Autodesk Inventor part; units mm, degrees
(part 4 of 5)
  spline S23 degree 5 poles (4.4219, -3.499) (4.422, -3.499) (4.4221, -3.4991) (4.4222, -3.4992) (4.4225, -3.4994) (4.423, -3.4998) (4.4234, -3.5001) (4.424, -3.5005) (4.4246, -3.501) (4.4253, -3.5015) (4.426, -3.502) (4.4268, -3.5026) (4.4277, -3.5032) (4.4286, -3.5039) (4.4296, -3.5046) (4.4307, -3.5053) (4.4318, -3.5061) (4.433, -3.5069) (4.4342, -3.5077) (4.4355, -3.5086) (4.4369, -3.5095) (4.4383, -3.5104) (4.4398, -3.5114) (4.4413, -3.5124) (4.4429, -3.5135) (4.4446, -3.5145) (4.4463, -3.5156) (4.4481, -3.5168) (4.4499, -3.5179) (4.4518, -3.5191) (4.4538, -3.5203) (4.4558, -3.5215) (4.4583, -3.5231) (4.4609, -3.5246) (4.4635, -3.5262) (4.4667, -3.5281) (4.4701, -3.53) (4.473, -3.5317) (4.4765, -3.5337) (4.4802, -3.5358) (4.4834, -3.5376) (4.4867, -3.5394) (4.4906, -3.5416) (4.4958, -3.5444) (4.5012, -3.5473) (4.5068, -3.5502) (4.5125, -3.5532) (4.5185, -3.5562) (4.5232, -3.5586) (4.528, -3.561) (4.533, -3.5635) (4.5387, -3.5663) (4.5439, -3.5687) (4.5484, -3.5709) (4.5538, -3.5734) (4.5592, -3.5759) (4.564, -3.5781) (4.5696, -3.5807) (4.5753, -3.5832) (4.5803, -3.5855) (4.5862, -3.5881) (4.5923, -3.5907) (4.5975, -3.5929) (4.6037, -3.5955) (4.61, -3.5982) (4.6155, -3.6004) (4.6219, -3.6031) (4.6285, -3.6057) (4.6342, -3.608) (4.641, -3.6107) (4.6478, -3.6133) (4.6537, -3.6156) (4.6607, -3.6183) (4.6679, -3.6209) (4.674, -3.6232) (4.6813, -3.6259) (4.6887, -3.6285) (4.6951, -3.6308) (4.7026, -3.6335) (4.7102, -3.6361) (4.7168, -3.6384) (4.7246, -3.641) (4.7325, -3.6437) (4.7393, -3.6459) (4.7474, -3.6485) (4.7555, -3.6511) (4.7626, -3.6533) (4.7708, -3.6559) (4.7792, -3.6585) (4.7865, -3.6607) (4.795, -3.6632) (4.8036, -3.6658) (4.8111, -3.6679) (4.8199, -3.6705) (4.8288, -3.6729) (4.8364, -3.6751) (4.8454, -3.6775) (4.8545, -3.68) (4.8624, -3.6821) (4.8717, -3.6845) (4.881, -3.6869) (4.8891, -3.6889) (4.8985, -3.6912) (4.9081, -3.6936) (4.9164, -3.6956) (4.9261, -3.6978) (4.9359, -3.7001) (4.9443, -3.702) (4.9543, -3.7043) (4.9643, -3.7065) (4.9729, -3.7083) (4.9831, -3.7105) (4.9933, -3.7126) (5.0021, -3.7144) (5.0125, -3.7165) (5.023, -3.7185) (5.032, -3.7202) (5.0425, -3.7222) (5.0532, -3.7242) (5.0624, -3.7258) (5.0732, -3.7277) (5.0841, -3.7296) (5.0934, -3.7312) (5.1044, -3.733) (5.1155, -3.7348) (5.1251, -3.7363) (5.1363, -3.738) (5.1475, -3.7397) (5.1572, -3.7411) (5.1686, -3.7427) (5.1801, -3.7443) (5.19, -3.7456) (5.2016, -3.7472) (5.2133, -3.7486) (5.2233, -3.7499) (5.2351, -3.7513) (5.247, -3.7527) (5.2572, -3.7538) (5.2692, -3.7551) (5.2812, -3.7564) (5.2916, -3.7574) (5.3037, -3.7586) (5.316, -3.7598) (5.3265, -3.7607) (5.3388, -3.7618) (5.3513, -3.7628) (5.3619, -3.7637) (5.3763, -3.7648) (5.3907, -3.7658) (5.4033, -3.7667) (5.4161, -3.7675) (5.4289, -3.7682) (5.4435, -3.7691) (5.4583, -3.7698) (5.4731, -3.7705) (5.4881, -3.7712) (5.505, -3.7718) (5.5163, -3.7722) (5.5276, -3.7726) (5.5428, -3.773) (5.5581, -3.7734) (5.5715, -3.7736) (5.585, -3.7738) (5.5985, -3.774) (5.6082, -3.7741) (5.6179, -3.7741) (5.6277, -3.7742) (5.6375, -3.7742) (5.6473, -3.7742) (5.6571, -3.7742) (5.667, -3.7741) (5.6769, -3.774) (5.6868, -3.7739) (5.6967, -3.7738) (5.7067, -3.7736) (5.7167, -3.7734) (5.7267, -3.7732) (5.7368, -3.7729) (5.7468, -3.7727) (5.757, -3.7724) (5.7671, -3.772) (5.7772, -3.7717) (5.7874, -3.7713) (5.7976, -3.7709) (5.8079, -3.7705) (5.8181, -3.77) (5.8284, -3.7695) (5.8387, -3.769) (5.849, -3.7685) (5.8635, -3.7677) (5.876, -3.7669) (5.8864, -3.7663) (5.8948, -3.7657) (5.901, -3.7653) knots 0 0 0 0 0 0 0.004167 0.008333 0.0125 0.016667 0.020833 0.025 0.029167 0.033333 0.0375 0.041667 0.045833 0.05 0.054167 0.058333 0.0625 0.066667 0.070833 0.075 0.079167 0.083333 0.0875 0.091667 0.095833 0.1 0.104167 0.108333 0.1125 0.116667 0.120833 0.125 0.129167 0.1375 0.141667 0.145833 0.154167 0.158333 0.1625 0.170833 0.175 0.179167 0.183333 0.191667 0.208333 0.2125 0.216667 0.220833 0.229167 0.2375 0.241667 0.245833 0.254167 0.258333 0.2625 0.270833 0.275 0.279167 0.2875 0.291667 0.295833 0.304167 0.308333 0.3125 0.320833 0.325 0.329167 0.3375 0.341667 0.345833 0.354167 0.358333 0.3625 0.370833 0.375 0.379167 0.3875 0.391667 0.395833 0.404167 0.408333 0.4125 0.420833 0.425 0.429167 0.4375 0.441667 0.445833 0.454167 0.458333 0.4625 0.470833 0.475 0.479167 0.4875 0.491667 0.495833 0.504167 0.508333 0.5125 0.520833 0.525 0.529167 0.5375 0.541667 0.545833 0.554167 0.558333 0.5625 0.570833 0.575 0.579167 0.5875 0.591667 0.595833 0.604167 0.608333 0.6125 0.620833 0.625 0.629167 0.6375 0.641667 0.645833 0.654167 0.658333 0.6625 0.670833 0.675 0.679167 0.6875 0.691667 0.695833 0.704167 0.708333 0.7125 0.720833 0.725 0.729167 0.7375 0.741667 0.745833 0.754167 0.758333 0.7625 0.770833 0.775 0.779167 0.791667 0.795833 0.8 0.804167 0.808333 0.825 0.829167 0.833333 0.8375 0.845833 0.85 0.854167 0.866667 0.870833 0.875 0.879167 0.883333 0.8875 0.891667 0.895833 0.9 0.904167 0.908333 0.9125 0.916667 0.920833 0.925 0.929167 0.933333 0.9375 0.941667 0.945833 0.95 0.954167 0.958333 0.9625 0.966667 0.970833 0.975 0.979167 0.983333 0.9875 1 1 1 1 1 1
  arc A23 (5.901, -3.7653) -> (6.2114, -3.2278) centre (0, 0) ccw
  circle A24 centre (0, 0) radius 3 construction
  line L24 (-4.4832, 3.4199) -> (-3.7077, 2.8063)
  arc A25 (-2.8063, 3.7077) -> (-3.7077, 2.8063) centre (0, 0) ccw
  line L25 (-2.8063, 3.7077) -> (-3.4199, 4.4832)
  arc A26 (-3.2267, 6.0991) -> (-3.6686, 5.8439) centre (0, 0) ccw
  line L26 (-2.1726, 5.2033) -> (-1.8078, 4.2842)
  arc A27 (-0.5765, 4.6141) -> (-1.8078, 4.2842) centre (0, 0) ccw
  line L27 (-0.5765, 4.6141) -> (-0.7202, 5.5925)
  arc A28 (0.2551, 6.8953) -> (-0.2551, 6.8953) centre (0, 0) ccw
  line L28 (0.7202, 5.5925) -> (0.5765, 4.6141)
  arc A29 (1.8078, 4.2842) -> (0.5765, 4.6141) centre (0, 0) ccw
  line L29 (1.8078, 4.2842) -> (2.1726, 5.2033)
  arc A30 (3.6686, 5.8439) -> (3.2267, 6.0991) centre (0, 0) ccw
  line L30 (3.4199, 4.4832) -> (2.8063, 3.7077)
  arc A31 (3.7077, 2.8063) -> (2.8063, 3.7077) centre (0, 0) ccw
  line L31 (3.7077, 2.8063) -> (4.4832, 3.4199)
  arc A32 (6.0991, 3.2267) -> (5.8439, 3.6686) centre (0, 0) ccw
  line L32 (5.2033, 2.1726) -> (4.2842, 1.8078)
  arc A33 (4.6141, 0.5765) -> (4.2842, 1.8078) centre (0, 0) ccw
  line L33 (4.6141, 0.5765) -> (5.5925, 0.7202)
  arc A34 (6.8953, -0.2551) -> (6.8953, 0.2551) centre (0, 0) ccw
  line L34 (5.5925, -0.7202) -> (4.6141, -0.5765)
  arc A35 (4.2842, -1.8078) -> (4.6141, -0.5765) centre (0, 0) ccw
  line L35 (4.2842, -1.8078) -> (5.2033, -2.1726)
  arc A36 (5.8439, -3.6686) -> (6.0991, -3.2267) centre (0, 0) ccw
  line L36 (4.4832, -3.4199) -> (3.7077, -2.8063)
  arc A37 (2.8063, -3.7077) -> (3.7077, -2.8063) centre (0, 0) ccw
  line L37 (2.8063, -3.7077) -> (3.4199, -4.4832)
  arc A38 (3.2267, -6.0991) -> (3.6686, -5.8439) centre (0, 0) ccw
  line L38 (2.1726, -5.2033) -> (1.8078, -4.2842)
  arc A39 (0.5765, -4.6141) -> (1.8078, -4.2842) centre (0, 0) ccw
  line L39 (0.5765, -4.6141) -> (0.7202, -5.5925)
  arc A40 (-0.2551, -6.8953) -> (0.2551, -6.8953) centre (0, 0) ccw
  line L40 (-0.7202, -5.5925) -> (-0.5765, -4.6141)
  arc A41 (-1.8078, -4.2842) -> (-0.5765, -4.6141) centre (0, 0) ccw
  line L41 (-1.8078, -4.2842) -> (-2.1726, -5.2033)
  arc A42 (-3.6686, -5.8439) -> (-3.2267, -6.0991) centre (0, 0) ccw
  line L42 (-3.4199, -4.4832) -> (-2.8063, -3.7077)
  arc A43 (-3.7077, -2.8063) -> (-2.8063, -3.7077) centre (0, 0) ccw
  line L43 (-3.7077, -2.8063) -> (-4.4832, -3.4199)
  arc A44 (-6.0991, -3.2267) -> (-5.8439, -3.6686) centre (0, 0) ccw
  line L44 (-5.2033, -2.1726) -> (-4.2842, -1.8078)
  arc A45 (-4.6141, -0.5765) -> (-4.2842, -1.8078) centre (0, 0) ccw
  line L45 (-4.6141, -0.5765) -> (-5.5925, -0.7202)
  arc A46 (-6.8953, 0.2551) -> (-6.8953, -0.2551) centre (0, 0) ccw
  line L46 (-5.5925, 0.7202) -> (-4.6141, 0.5765)
  arc A47 (-4.2842, 1.8078) -> (-4.6141, 0.5765) centre (0, 0) ccw
  line L47 (-4.2842, 1.8078) -> (-5.2033, 2.1726)
  arc A48 (-5.8439, 3.6686) -> (-6.0991, 3.2267) centre (0, 0) ccw
  line L48 (-0.5765, 4.6141) -> (0.5765, 4.6141) construction
  spline S24 degree 5 poles (-3.4199, 4.4832) (-3.4189, 4.4818) (-3.4217, 4.4856) (-3.4213, 4.485) (-3.4244, 4.4895) (-3.4266, 4.4928) (-3.4288, 4.496) (-3.4335, 4.5035) (-3.4383, 4.5113) (-3.4411, 4.5161) (-3.4477, 4.5274) (-3.454, 4.5388) (-3.4576, 4.5454) (-3.4654, 4.5602) (-3.4728, 4.5752) (-3.4769, 4.5835) (-3.4855, 4.6017) (-3.4937, 4.62) (-3.4981, 4.63) (-3.5072, 4.6514) (-3.5159, 4.673) (-3.5204, 4.6845) (-3.5297, 4.709) (-3.5385, 4.7337) (-3.543, 4.7467) (-3.5522, 4.7741) (-3.5609, 4.8017) (-3.5653, 4.8162) (-3.5742, 4.8465) (-3.5825, 4.8769) (-3.5867, 4.8927) (-3.5951, 4.9256) (-3.6028, 4.9587) (-3.6067, 4.9758) (-3.6144, 5.0113) (-3.6214, 5.0469) (-3.6248, 5.0653) (-3.6316, 5.1033) (-3.6377, 5.1413) (-3.6407, 5.1609) (-3.6464, 5.2011) (-3.6514, 5.2414) (-3.6538, 5.2621) (-3.6584, 5.3045) (-3.6622, 5.347) (-3.664, 5.3688) (-3.6673, 5.4132) (-3.6698, 5.4578) (-3.6708, 5.4805) (-3.6727, 5.527) (-3.6737, 5.5734) (-3.6741, 5.5971) (-3.6744, 5.6454) (-3.6739, 5.6937) (-3.6735, 5.7183) (-3.6724, 5.7581) (-3.6708, 5.798) (-3.6702, 5.8133) (-3.6694, 5.8286) (-3.6686, 5.8439) knots 0 0 0 0 0 0 0.004377 0.004377 0.004377 0.016733 0.016733 0.016733 0.036594 0.036594 0.036594 0.063277 0.063277 0.063277 0.096218 0.096218 0.096218 0.134948 0.134948 0.134948 0.179064 0.179064 0.179064 0.228222 0.228222 0.228222 0.282124 0.282124 0.282124 0.340507 0.340507 0.340507 0.403138 0.403138 0.403138 0.46981 0.46981 0.46981 0.540337 0.540337 0.540337 0.614551 0.614551 0.614551 0.692299 0.692299 0.692299 0.773444 0.773444 0.773444 0.857857 0.857857 0.857857 0.945422 0.945422 0.945422 1 1 1 1 1 1
  spline S25 degree 5 poles (-3.2267, 6.0991) (-3.213, 6.0921) (-3.1994, 6.0851) (-3.1858, 6.078) (-3.1505, 6.0595) (-3.1154, 6.0404) (-3.0939, 6.0285) (-3.0519, 6.0048) (-3.0102, 5.9804) (-2.9899, 5.9683) (-2.9502, 5.9441) (-2.9109, 5.9193) (-2.8917, 5.907) (-2.8544, 5.8826) (-2.8175, 5.8575) (-2.7995, 5.8451) (-2.7646, 5.8205) (-2.7302, 5.7954) (-2.7135, 5.7829) (-2.6811, 5.7584) (-2.6491, 5.7333) (-2.6336, 5.721) (-2.6037, 5.6967) (-2.5743, 5.6719) (-2.5601, 5.6597) (-2.5328, 5.6358) (-2.5059, 5.6114) (-2.4929, 5.5995) (-2.4682, 5.5762) (-2.4439, 5.5525) (-2.4322, 5.541) (-2.4101, 5.5186) (-2.3883, 5.4957) (-2.378, 5.4847) (-2.3584, 5.4634) (-2.3393, 5.4417) (-2.3302, 5.4312) (-2.3133, 5.4113) (-2.2967, 5.391) (-2.289, 5.3813) (-2.2746, 5.363) (-2.2607, 5.3444) (-2.2542, 5.3357) (-2.2424, 5.3194) (-2.231, 5.3028) (-2.2258, 5.2952) (-2.2166, 5.2812) (-2.2077, 5.2671) (-2.2037, 5.2607) (-2.197, 5.2495) (-2.1905, 5.2381) (-2.1878, 5.2334) (-2.1834, 5.2252) (-2.1793, 5.2174) (-2.1776, 5.2139) (-2.1758, 5.2104) (-2.1735, 5.2054) (-2.1738, 5.2061) (-2.1719, 5.2017) (-2.1726, 5.2033) knots 0 0 0 0 0 0 0.054578 0.054578 0.054578 0.142143 0.142143 0.142143 0.226556 0.226556 0.226556 0.307701 0.307701 0.307701 0.385449 0.385449 0.385449 0.459663 0.459663 0.459663 0.53019 0.53019 0.53019 0.596862 0.596862 0.596862 0.659493 0.659493 0.659493 0.717876 0.717876 0.717876 0.771778 0.771778 0.771778 0.820936 0.820936 0.820936 0.865052 0.865052 0.865052 0.903782 0.903782 0.903782 0.936723 0.936723 0.936723 0.963406 0.963406 0.963406 0.983267 0.983267 0.983267 0.995623 0.995623 0.995623 1 1 1 1 1 1
  spline S26 degree 5 poles (-0.7202, 5.5925) (-0.7199, 5.5908) (-0.7205, 5.5955) (-0.7204, 5.5948) (-0.7209, 5.6002) (-0.7211, 5.6042) (-0.7214, 5.6081) (-0.7218, 5.6169) (-0.722, 5.6261) (-0.7221, 5.6316) (-0.7221, 5.6447) (-0.7219, 5.6577) (-0.7216, 5.6652) (-0.721, 5.6819) (-0.72, 5.6987) (-0.7193, 5.7079) (-0.7177, 5.7279) (-0.7157, 5.7479) (-0.7144, 5.7588) (-0.7116, 5.7818) (-0.7083, 5.8049) (-0.7065, 5.8171) (-0.7023, 5.843) (-0.6976, 5.8687) (-0.695, 5.8823) (-0.6892, 5.9106) (-0.683, 5.9389) (-0.6795, 5.9536) (-0.6721, 5.9842) (-0.6641, 6.0147) (-0.6598, 6.0306) (-0.6506, 6.0632) (-0.6408, 6.0958) (-0.6356, 6.1126) (-0.6245, 6.1471) (-0.6127, 6.1815) (-0.6065, 6.1991) (-0.5934, 6.2353) (-0.5797, 6.2713) (-0.5725, 6.2898) (-0.5573, 6.3275) (-0.5415, 6.3649) (-0.5333, 6.384) (-0.516, 6.423) (-0.4981, 6.4618) (-0.4887, 6.4815) (-0.4693, 6.5216) (-0.4492, 6.5615) (-0.4388, 6.5817) (-0.4172, 6.6228) (-0.3948, 6.6636) (-0.3833, 6.6843) (-0.3594, 6.7263) (-0.3349, 6.7678) (-0.3222, 6.7889) (-0.3013, 6.8229) (-0.28, 6.8567) (-0.2718, 6.8696) (-0.2635, 6.8824) (-0.2551, 6.8953) knots 0 0 0 0 0 0 0.004377 0.004377 0.004377 0.016733 0.016733 0.016733 0.036594 0.036594 0.036594 0.063277 0.063277 0.063277 0.096218 0.096218 0.096218 0.134948 0.134948 0.134948 0.179064 0.179064 0.179064 0.228222 0.228222 0.228222 0.282124 0.282124 0.282124 0.340507 0.340507 0.340507 0.403138 0.403138 0.403138 0.46981 0.46981 0.46981 0.540337 0.540337 0.540337 0.614551 0.614551 0.614551 0.692299 0.692299 0.692299 0.773444 0.773444 0.773444 0.857857 0.857857 0.857857 0.945422 0.945422 0.945422 1 1 1 1 1 1
  spline S27 degree 5 poles (0.2551, 6.8953) (0.2635, 6.8824) (0.2718, 6.8696) (0.28, 6.8567) (0.3013, 6.8229) (0.3222, 6.7889) (0.3349, 6.7678) (0.3594, 6.7263) (0.3833, 6.6843) (0.3948, 6.6636) (0.4172, 6.6228) (0.4388, 6.5817) (0.4492, 6.5615) (0.4693, 6.5216) (0.4887, 6.4815) (0.4981, 6.4618) (0.516, 6.423) (0.5333, 6.384) (0.5415, 6.3649) (0.5573, 6.3275) (0.5725, 6.2898) (0.5797, 6.2713) (0.5934, 6.2353) (0.6065, 6.1991) (0.6127, 6.1815) (0.6245, 6.1471) (0.6356, 6.1126) (0.6408, 6.0958) (0.6506, 6.0632) (0.6598, 6.0306) (0.6641, 6.0147) (0.6721, 5.9842) (0.6795, 5.9536) (0.683, 5.9389) (0.6892, 5.9106) (0.695, 5.8823) (0.6976, 5.8687) (0.7023, 5.843) (0.7065, 5.8171) (0.7083, 5.8049) (0.7116, 5.7818) (0.7144, 5.7588) (0.7157, 5.7479) (0.7177, 5.7279) (0.7193, 5.7079) (0.72, 5.6987) (0.721, 5.6819) (0.7216, 5.6652) (0.7219, 5.6577) (0.7221, 5.6447) (0.7221, 5.6316) (0.722, 5.6261) (0.7218, 5.6169) (0.7214, 5.6081) (0.7211, 5.6042) (0.7209, 5.6002) (0.7204, 5.5948) (0.7205, 5.5955) (0.7199, 5.5908) (0.7202, 5.5925) knots 0 0 0 0 0 0 0.054578 0.054578 0.054578 0.142143 0.142143 0.142143 0.226556 0.226556 0.226556 0.307701 0.307701 0.307701 0.385449 0.385449 0.385449 0.459663 0.459663 0.459663 0.53019 0.53019 0.53019 0.596862 0.596862 0.596862 0.659493 0.659493 0.659493 0.717876 0.717876 0.717876 0.771778 0.771778 0.771778 0.820936 0.820936 0.820936 0.865052 0.865052 0.865052 0.903782 0.903782 0.903782 0.936723 0.936723 0.936723 0.963406 0.963406 0.963406 0.983267 0.983267 0.983267 0.995623 0.995623 0.995623 1 1 1 1 1 1
  spline S28 degree 5 poles (2.1726, 5.2033) (2.1719, 5.2017) (2.1738, 5.2061) (2.1735, 5.2054) (2.1758, 5.2104) (2.1776, 5.2139) (2.1793, 5.2174) (2.1834, 5.2252) (2.1878, 5.2334) (2.1905, 5.2381) (2.197, 5.2495) (2.2037, 5.2607) (2.2077, 5.2671) (2.2166, 5.2812) (2.2258, 5.2952) (2.231, 5.3028) (2.2424, 5.3194) (2.2542, 5.3357) (2.2607, 5.3444) (2.2746, 5.363) (2.289, 5.3813) (2.2967, 5.391) (2.3133, 5.4113) (2.3302, 5.4312) (2.3393, 5.4417) (2.3584, 5.4634) (2.378, 5.4847) (2.3883, 5.4957) (2.4101, 5.5186) (2.4322, 5.541) (2.4439, 5.5525) (2.4682, 5.5762) (2.4929, 5.5995) (2.5059, 5.6114) (2.5328, 5.6358) (2.5601, 5.6597) (2.5743, 5.6719) (2.6037, 5.6967) (2.6336, 5.721) (2.6491, 5.7333) (2.6811, 5.7584) (2.7135, 5.7829) (2.7302, 5.7954) (2.7646, 5.8205) (2.7995, 5.8451) (2.8175, 5.8575) (2.8544, 5.8826) (2.8917, 5.907) (2.9109, 5.9193) (2.9502, 5.9441) (2.9899, 5.9683) (3.0102, 5.9804) (3.0519, 6.0048) (3.0939, 6.0285) (3.1154, 6.0404) (3.1505, 6.0595) (3.1858, 6.078) (3.1994, 6.0851) (3.213, 6.0921) (3.2267, 6.0991) knots 0 0 0 0 0 0 0.004377 0.004377 0.004377 0.016733 0.016733 0.016733 0.036594 0.036594 0.036594 0.063277 0.063277 0.063277 0.096218 0.096218 0.096218 0.134948 0.134948 0.134948 0.179064 0.179064 0.179064 0.228222 0.228222 0.228222 0.282124 0.282124 0.282124 0.340507 0.340507 0.340507 0.403138 0.403138 0.403138 0.46981 0.46981 0.46981 0.540337 0.540337 0.540337 0.614551 0.614551 0.614551 0.692299 0.692299 0.692299 0.773444 0.773444 0.773444 0.857857 0.857857 0.857857 0.945422 0.945422 0.945422 1 1 1 1 1 1
  spline S29 degree 5 poles (3.6686, 5.8439) (3.6694, 5.8286) (3.6702, 5.8133) (3.6708, 5.798) (3.6724, 5.7581) (3.6735, 5.7183) (3.6739, 5.6937) (3.6744, 5.6454) (3.6741, 5.5971) (3.6737, 5.5734) (3.6727, 5.527) (3.6708, 5.4805) (3.6698, 5.4578) (3.6673, 5.4132) (3.664, 5.3688) (3.6622, 5.347) (3.6584, 5.3045) (3.6538, 5.2621) (3.6514, 5.2414) (3.6464, 5.2011) (3.6407, 5.1609) (3.6377, 5.1413) (3.6316, 5.1033) (3.6248, 5.0653) (3.6214, 5.0469) (3.6144, 5.0113) (3.6067, 4.9758) (3.6028, 4.9587) (3.5951, 4.9256) (3.5867, 4.8927) (3.5825, 4.8769) (3.5742, 4.8465) (3.5653, 4.8162) (3.5609, 4.8017) (3.5522, 4.7741) (3.543, 4.7467) (3.5385, 4.7337) (3.5297, 4.709) (3.5204, 4.6845) (3.5159, 4.673) (3.5072, 4.6514) (3.4981, 4.63) (3.4937, 4.62) (3.4855, 4.6017) (3.4769, 4.5835) (3.4728, 4.5752) (3.4654, 4.5602) (3.4576, 4.5454) (3.454, 4.5388) (3.4477, 4.5274) (3.4411, 4.5161) (3.4383, 4.5113) (3.4335, 4.5035) (3.4288, 4.496) (3.4266, 4.4928) (3.4244, 4.4895) (3.4213, 4.485) (3.4217, 4.4856) (3.4189, 4.4818) (3.4199, 4.4832) knots 0 0 0 0 0 0 0.054578 0.054578 0.054578 0.142143 0.142143 0.142143 0.226556 0.226556 0.226556 0.307701 0.307701 0.307701 0.385449 0.385449 0.385449 0.459663 0.459663 0.459663 0.53019 0.53019 0.53019 0.596862 0.596862 0.596862 0.659493 0.659493 0.659493 0.717875 0.717875 0.717875 0.771778 0.771778 0.771778 0.820936 0.820936 0.820936 0.865052 0.865052 0.865052 0.903781 0.903781 0.903781 0.936723 0.936723 0.936723 0.963406 0.963406 0.963406 0.983267 0.983267 0.983267 0.995622 0.995622 0.995622 1 1 1 1 1 1
  spline S30 degree 5 poles (4.4832, 3.4199) (4.4818, 3.4189) (4.4856, 3.4217) (4.485, 3.4213) (4.4895, 3.4244) (4.4928, 3.4266) (4.496, 3.4288) (4.5035, 3.4335) (4.5113, 3.4383) (4.5161, 3.4411) (4.5274, 3.4477) (4.5388, 3.454) (4.5454, 3.4576) (4.5602, 3.4654) (4.5752, 3.4728) (4.5835, 3.4769) (4.6017, 3.4855) (4.62, 3.4937) (4.63, 3.4981) (4.6514, 3.5072) (4.673, 3.5159) (4.6845, 3.5204) (4.709, 3.5297) (4.7337, 3.5385) (4.7467, 3.543) (4.7741, 3.5522) (4.8017, 3.5609) (4.8162, 3.5653) (4.8465, 3.5742) (4.8769, 3.5825) (4.8927, 3.5867) (4.9256, 3.5951) (4.9587, 3.6028) (4.9758, 3.6067) (5.0113, 3.6144) (5.0469, 3.6214) (5.0653, 3.6248) (5.1033, 3.6316) (5.1413, 3.6377) (5.1609, 3.6407) (5.2011, 3.6464) (5.2414, 3.6514) (5.2621, 3.6538) (5.3045, 3.6584) (5.347, 3.6622) (5.3688, 3.664) (5.4132, 3.6673) (5.4578, 3.6698) (5.4805, 3.6708) (5.527, 3.6727) (5.5734, 3.6737) (5.5971, 3.6741) (5.6454, 3.6744) (5.6937, 3.6739) (5.7183, 3.6735) (5.7581, 3.6724) (5.798, 3.6708) (5.8133, 3.6702) (5.8286, 3.6694) (5.8439, 3.6686) knots 0 0 0 0 0 0 0.004377 0.004377 0.004377 0.016733 0.016733 0.016733 0.036594 0.036594 0.036594 0.063277 0.063277 0.063277 0.096218 0.096218 0.096218 0.134948 0.134948 0.134948 0.179064 0.179064 0.179064 0.228222 0.228222 0.228222 0.282124 0.282124 0.282124 0.340507 0.340507 0.340507 0.403138 0.403138 0.403138 0.46981 0.46981 0.46981 0.540337 0.540337 0.540337 0.614551 0.614551 0.614551 0.692299 0.692299 0.692299 0.773444 0.773444 0.773444 0.857857 0.857857 0.857857 0.945422 0.945422 0.945422 1 1 1 1 1 1
  spline S31 degree 5 poles (6.0991, 3.2267) (6.0921, 3.213) (6.0851, 3.1994) (6.078, 3.1858) (6.0595, 3.1505) (6.0404, 3.1154) (6.0285, 3.0939) (6.0048, 3.0519) (5.9804, 3.0102) (5.9683, 2.9899) (5.9441, 2.9502) (5.9193, 2.9109) (5.907, 2.8917) (5.8826, 2.8544) (5.8575, 2.8175) (5.8451, 2.7995) (5.8205, 2.7646) (5.7954, 2.7302) (5.7829, 2.7135) (5.7584, 2.6811) (5.7333, 2.6491) (5.721, 2.6336) (5.6967, 2.6037) (5.6719, 2.5743) (5.6597, 2.5601) (5.6358, 2.5328) (5.6114, 2.5059) (5.5995, 2.4929) (5.5762, 2.4682) (5.5525, 2.4439) (5.541, 2.4322) (5.5186, 2.4101) (5.4957, 2.3883) (5.4847, 2.378) (5.4634, 2.3584) (5.4417, 2.3393) (5.4312, 2.3302) (5.4113, 2.3133) (5.391, 2.2967) (5.3813, 2.289) (5.363, 2.2746) (5.3444, 2.2607) (5.3357, 2.2542) (5.3194, 2.2424) (5.3028, 2.231) (5.2952, 2.2258) (5.2812, 2.2166) (5.2671, 2.2077) (5.2607, 2.2037) (5.2495, 2.197) (5.2381, 2.1905) (5.2334, 2.1878) (5.2252, 2.1834) (5.2174, 2.1793) (5.2139, 2.1776) (5.2104, 2.1758) (5.2054, 2.1735) (5.2061, 2.1738) (5.2017, 2.1719) (5.2033, 2.1726) knots 0 0 0 0 0 0 0.054578 0.054578 0.054578 0.142143 0.142143 0.142143 0.226556 0.226556 0.226556 0.307701 0.307701 0.307701 0.385449 0.385449 0.385449 0.459663 0.459663 0.459663 0.53019 0.53019 0.53019 0.596862 0.596862 0.596862 0.659493 0.659493 0.659493 0.717876 0.717876 0.717876 0.771778 0.771778 0.771778 0.820936 0.820936 0.820936 0.865052 0.865052 0.865052 0.903782 0.903782 0.903782 0.936723 0.936723 0.936723 0.963406 0.963406 0.963406 0.983267 0.983267 0.983267 0.995623 0.995623 0.995623 1 1 1 1 1 1
  spline S32 degree 5 poles (5.5925, 0.7202) (5.5908, 0.7199) (5.5955, 0.7205) (5.5948, 0.7204) (5.6002, 0.7209) (5.6042, 0.7211) (5.6081, 0.7214) (5.6169, 0.7218) (5.6261, 0.722) (5.6316, 0.7221) (5.6447, 0.7221) (5.6577, 0.7219) (5.6652, 0.7216) (5.6819, 0.721) (5.6987, 0.72) (5.7079, 0.7193) (5.7279, 0.7177) (5.7479, 0.7157) (5.7588, 0.7144) (5.7818, 0.7116) (5.8049, 0.7083) (5.8171, 0.7065) (5.843, 0.7023) (5.8687, 0.6976) (5.8823, 0.695) (5.9106, 0.6892) (5.9389, 0.683) (5.9536, 0.6795) (5.9842, 0.6721) (6.0147, 0.6641) (6.0306, 0.6598) (6.0632, 0.6506) (6.0958, 0.6408) (6.1126, 0.6356) (6.1471, 0.6245) (6.1815, 0.6127) (6.1991, 0.6065) (6.2353, 0.5934) (6.2713, 0.5797) (6.2898, 0.5725) (6.3275, 0.5573) (6.3649, 0.5415) (6.384, 0.5333) (6.423, 0.516) (6.4618, 0.4981) (6.4815, 0.4887) (6.5216, 0.4693) (6.5615, 0.4492) (6.5817, 0.4388) (6.6228, 0.4172) (6.6636, 0.3948) (6.6843, 0.3833) (6.7263, 0.3594) (6.7678, 0.3349) (6.7889, 0.3222) (6.8229, 0.3013) (6.8567, 0.28) (6.8696, 0.2718) (6.8824, 0.2635) (6.8953, 0.2551) knots 0 0 0 0 0 0 0.004377 0.004377 0.004377 0.016733 0.016733 0.016733 0.036594 0.036594 0.036594 0.063277 0.063277 0.063277 0.096218 0.096218 0.096218 0.134948 0.134948 0.134948 0.179064 0.179064 0.179064 0.228222 0.228222 0.228222 0.282124 0.282124 0.282124 0.340507 0.340507 0.340507 0.403138 0.403138 0.403138 0.46981 0.46981 0.46981 0.540337 0.540337 0.540337 0.614551 0.614551 0.614551 0.692299 0.692299 0.692299 0.773444 0.773444 0.773444 0.857857 0.857857 0.857857 0.945422 0.945422 0.945422 1 1 1 1 1 1
  spline S33 degree 5 poles (6.8953, -0.2551) (6.8824, -0.2635) (6.8696, -0.2718) (6.8567, -0.28) (6.8229, -0.3013) (6.7889, -0.3222) (6.7678, -0.3349) (6.7263, -0.3594) (6.6843, -0.3833) (6.6636, -0.3948) (6.6228, -0.4172) (6.5817, -0.4388) (6.5615, -0.4492) (6.5216, -0.4693) (6.4815, -0.4887) (6.4618, -0.4981) (6.423, -0.516) (6.384, -0.5333) (6.3649, -0.5415) (6.3275, -0.5573) (6.2898, -0.5725) (6.2713, -0.5797) (6.2353, -0.5934) (6.1991, -0.6065) (6.1815, -0.6127) (6.1471, -0.6245) (6.1126, -0.6356) (6.0958, -0.6408) (6.0632, -0.6506) (6.0306, -0.6598) (6.0147, -0.6641) (5.9842, -0.6721) (5.9536, -0.6795) (5.9389, -0.683) (5.9106, -0.6892) (5.8823, -0.695) (5.8687, -0.6976) (5.843, -0.7023) (5.8171, -0.7065) (5.8049, -0.7083) (5.7818, -0.7116) (5.7588, -0.7144) (5.7479, -0.7157) (5.7279, -0.7177) (5.7079, -0.7193) (5.6987, -0.72) (5.6819, -0.721) (5.6652, -0.7216) (5.6577, -0.7219) (5.6447, -0.7221) (5.6316, -0.7221) (5.6261, -0.722) (5.6169, -0.7218) (5.6081, -0.7214) (5.6042, -0.7211) (5.6002, -0.7209) (5.5948, -0.7204) (5.5955, -0.7205) (5.5908, -0.7199) (5.5925, -0.7202) knots 0 0 0 0 0 0 0.054578 0.054578 0.054578 0.142143 0.142143 0.142143 0.226556 0.226556 0.226556 0.307701 0.307701 0.307701 0.385449 0.385449 0.385449 0.459663 0.459663 0.459663 0.53019 0.53019 0.53019 0.596862 0.596862 0.596862 0.659493 0.659493 0.659493 0.717876 0.717876 0.717876 0.771778 0.771778 0.771778 0.820936 0.820936 0.820936 0.865052 0.865052 0.865052 0.903782 0.903782 0.903782 0.936723 0.936723 0.936723 0.963406 0.963406 0.963406 0.983267 0.983267 0.983267 0.995623 0.995623 0.995623 1 1 1 1 1 1
  spline S34 degree 5 poles (5.2033, -2.1726) (5.2017, -2.1719) (5.2061, -2.1738) (5.2054, -2.1735) (5.2104, -2.1758) (5.2139, -2.1776) (5.2174, -2.1793) (5.2252, -2.1834) (5.2334, -2.1878) (5.2381, -2.1905) (5.2495, -2.197) (5.2607, -2.2037) (5.2671, -2.2077) (5.2812, -2.2166) (5.2952, -2.2258) (5.3028, -2.231) (5.3194, -2.2424) (5.3357, -2.2542) (5.3444, -2.2607) (5.363, -2.2746) (5.3813, -2.289) (5.391, -2.2967) (5.4113, -2.3133) (5.4312, -2.3302) (5.4417, -2.3393) (5.4634, -2.3584) (5.4847, -2.378) (5.4957, -2.3883) (5.5186, -2.4101) (5.541, -2.4322) (5.5525, -2.4439) (5.5762, -2.4682) (5.5995, -2.4929) (5.6114, -2.5059) (5.6358, -2.5328) (5.6597, -2.5601) (5.6719, -2.5743) (5.6967, -2.6037) (5.721, -2.6336) (5.7333, -2.6491) (5.7584, -2.6811) (5.7829, -2.7135) (5.7954, -2.7302) (5.8205, -2.7646) (5.8451, -2.7995) (5.8575, -2.8175) (5.8826, -2.8544) (5.907, -2.8917) (5.9193, -2.9109) (5.9441, -2.9502) (5.9683, -2.9899) (5.9804, -3.0102) (6.0048, -3.0519) (6.0285, -3.0939) (6.0404, -3.1154) (6.0595, -3.1505) (6.078, -3.1858) (6.0851, -3.1994) (6.0921, -3.213) (6.0991, -3.2267) knots 0 0 0 0 0 0 0.004377 0.004377 0.004377 0.016733 0.016733 0.016733 0.036594 0.036594 0.036594 0.063277 0.063277 0.063277 0.096218 0.096218 0.096218 0.134948 0.134948 0.134948 0.179064 0.179064 0.179064 0.228222 0.228222 0.228222 0.282124 0.282124 0.282124 0.340507 0.340507 0.340507 0.403138 0.403138 0.403138 0.46981 0.46981 0.46981 0.540337 0.540337 0.540337 0.614551 0.614551 0.614551 0.692299 0.692299 0.692299 0.773444 0.773444 0.773444 0.857857 0.857857 0.857857 0.945422 0.945422 0.945422 1 1 1 1 1 1
  spline S35 degree 5 poles (5.8439, -3.6686) (5.8286, -3.6694) (5.8133, -3.6702) (5.798, -3.6708) (5.7581, -3.6724) (5.7183, -3.6735) (5.6937, -3.6739) (5.6454, -3.6744) (5.5971, -3.6741) (5.5734, -3.6737) (5.527, -3.6727) (5.4805, -3.6708) (5.4578, -3.6698) (5.4132, -3.6673) (5.3688, -3.664) (5.347, -3.6622) (5.3045, -3.6584) (5.2621, -3.6538) (5.2414, -3.6514) (5.2011, -3.6464) (5.1609, -3.6407) (5.1413, -3.6377) (5.1033, -3.6316) (5.0653, -3.6248) (5.0469, -3.6214) (5.0113, -3.6144) (4.9758, -3.6067) (4.9587, -3.6028) (4.9256, -3.5951) (4.8927, -3.5867) (4.8769, -3.5825) (4.8465, -3.5742) (4.8162, -3.5653) (4.8017, -3.5609) (4.7741, -3.5522) (4.7467, -3.543) (4.7337, -3.5385) (4.709, -3.5297) (4.6845, -3.5204) (4.673, -3.5159) (4.6514, -3.5072) (4.63, -3.4981) (4.62, -3.4937) (4.6017, -3.4855) (4.5835, -3.4769) (4.5752, -3.4728) (4.5602, -3.4654) (4.5454, -3.4576) (4.5388, -3.454) (4.5274, -3.4477) (4.5161, -3.4411) (4.5113, -3.4383) (4.5035, -3.4335) (4.496, -3.4288) (4.4928, -3.4266) (4.4895, -3.4244) (4.485, -3.4213) (4.4856, -3.4217) (4.4818, -3.4189) (4.4832, -3.4199) knots 0 0 0 0 0 0 0.054578 0.054578 0.054578 0.142143 0.142143 0.142143 0.226556 0.226556 0.226556 0.307701 0.307701 0.307701 0.385449 0.385449 0.385449 0.459663 0.459663 0.459663 0.53019 0.53019 0.53019 0.596862 0.596862 0.596862 0.659493 0.659493 0.659493 0.717875 0.717875 0.717875 0.771778 0.771778 0.771778 0.820936 0.820936 0.820936 0.865052 0.865052 0.865052 0.903781 0.903781 0.903781 0.936723 0.936723 0.936723 0.963406 0.963406 0.963406 0.983267 0.983267 0.983267 0.995622 0.995622 0.995622 1 1 1 1 1 1
  spline S36 degree 5 poles (3.4199, -4.4832) (3.4189, -4.4818) (3.4217, -4.4856) (3.4213, -4.485) (3.4244, -4.4895) (3.4266, -4.4928) (3.4288, -4.496) (3.4335, -4.5035) (3.4383, -4.5113) (3.4411, -4.5161) (3.4477, -4.5274) (3.454, -4.5388) (3.4576, -4.5454) (3.4654, -4.5602) (3.4728, -4.5752) (3.4769, -4.5835) (3.4855, -4.6017) (3.4937, -4.62) (3.4981, -4.63) (3.5072, -4.6514) (3.5159, -4.673) (3.5204, -4.6845) (3.5297, -4.709) (3.5385, -4.7337) (3.543, -4.7467) (3.5522, -4.7741) (3.5609, -4.8017) (3.5653, -4.8162) (3.5742, -4.8465) (3.5825, -4.8769) (3.5867, -4.8927) (3.5951, -4.9256) (3.6028, -4.9587) (3.6067, -4.9758) (3.6144, -5.0113) (3.6214, -5.0469) (3.6248, -5.0653) (3.6316, -5.1033) (3.6377, -5.1413) (3.6407, -5.1609) (3.6464, -5.2011) (3.6514, -5.2414) (3.6538, -5.2621) (3.6584, -5.3045) (3.6622, -5.347) (3.664, -5.3688) (3.6673, -5.4132) (3.6698, -5.4578) (3.6708, -5.4805) (3.6727, -5.527) (3.6737, -5.5734) (3.6741, -5.5971) (3.6744, -5.6454) (3.6739, -5.6937) (3.6735, -5.7183) (3.6724, -5.7581) (3.6708, -5.798) (3.6702, -5.8133) (3.6694, -5.8286) (3.6686, -5.8439) knots 0 0 0 0 0 0 0.004377 0.004377 0.004377 0.016733 0.016733 0.016733 0.036594 0.036594 0.036594 0.063277 0.063277 0.063277 0.096218 0.096218 0.096218 0.134948 0.134948 0.134948 0.179064 0.179064 0.179064 0.228222 0.228222 0.228222 0.282124 0.282124 0.282124 0.340507 0.340507 0.340507 0.403138 0.403138 0.403138 0.46981 0.46981 0.46981 0.540337 0.540337 0.540337 0.614551 0.614551 0.614551 0.692299 0.692299 0.692299 0.773444 0.773444 0.773444 0.857857 0.857857 0.857857 0.945422 0.945422 0.945422 1 1 1 1 1 1
  spline S37 degree 5 poles (3.2267, -6.0991) (3.213, -6.0921) (3.1994, -6.0851) (3.1858, -6.078) (3.1505, -6.0595) (3.1154, -6.0404) (3.0939, -6.0285) (3.0519, -6.0048) (3.0102, -5.9804) (2.9899, -5.9683) (2.9502, -5.9441) (2.9109, -5.9193) (2.8917, -5.907) (2.8544, -5.8826) (2.8175, -5.8575) (2.7995, -5.8451) (2.7646, -5.8205) (2.7302, -5.7954) (2.7135, -5.7829) (2.6811, -5.7584) (2.6491, -5.7333) (2.6336, -5.721) (2.6037, -5.6967) (2.5743, -5.6719) (2.5601, -5.6597) (2.5328, -5.6358) (2.5059, -5.6114) (2.4929, -5.5995) (2.4682, -5.5762) (2.4439, -5.5525) (2.4322, -5.541) (2.4101, -5.5186) (2.3883, -5.4957) (2.378, -5.4847) (2.3584, -5.4634) (2.3393, -5.4417) (2.3302, -5.4312) (2.3133, -5.4113) (2.2967, -5.391) (2.289, -5.3813) (2.2746, -5.363) (2.2607, -5.3444) (2.2542, -5.3357) (2.2424, -5.3194) (2.231, -5.3028) (2.2258, -5.2952) (2.2166, -5.2812) (2.2077, -5.2671) (2.2037, -5.2607) (2.197, -5.2495) (2.1905, -5.2381) (2.1878, -5.2334) (2.1834, -5.2252) (2.1793, -5.2174) (2.1776, -5.2139) (2.1758, -5.2104) (2.1735, -5.2054) (2.1738, -5.2061) (2.1719, -5.2017) (2.1726, -5.2033) knots 0 0 0 0 0 0 0.054578 0.054578 0.054578 0.142143 0.142143 0.142143 0.226556 0.226556 0.226556 0.307701 0.307701 0.307701 0.385449 0.385449 0.385449 0.459663 0.459663 0.459663 0.53019 0.53019 0.53019 0.596862 0.596862 0.596862 0.659493 0.659493 0.659493 0.717876 0.717876 0.717876 0.771778 0.771778 0.771778 0.820936 0.820936 0.820936 0.865052 0.865052 0.865052 0.903782 0.903782 0.903782 0.936723 0.936723 0.936723 0.963406 0.963406 0.963406 0.983267 0.983267 0.983267 0.995623 0.995623 0.995623 1 1 1 1 1 1
  spline S38 degree 5 poles (0.7202, -5.5925) (0.7199, -5.5908) (0.7205, -5.5955) (0.7204, -5.5948) (0.7209, -5.6002) (0.7211, -5.6042) (0.7214, -5.6081) (0.7218, -5.6169) (0.722, -5.6261) (0.7221, -5.6316) (0.7221, -5.6447) (0.7219, -5.6577) (0.7216, -5.6652) (0.721, -5.6819) (0.72, -5.6987) (0.7193, -5.7079) (0.7177, -5.7279) (0.7157, -5.7479) (0.7144, -5.7588) (0.7116, -5.7818) (0.7083, -5.8049) (0.7065, -5.8171) (0.7023, -5.843) (0.6976, -5.8687) (0.695, -5.8823) (0.6892, -5.9106) (0.683, -5.9389) (0.6795, -5.9536) (0.6721, -5.9842) (0.6641, -6.0147) (0.6598, -6.0306) (0.6506, -6.0632) (0.6408, -6.0958) (0.6356, -6.1126) (0.6245, -6.1471) (0.6127, -6.1815) (0.6065, -6.1991) (0.5934, -6.2353) (0.5797, -6.2713) (0.5725, -6.2898) (0.5573, -6.3275) (0.5415, -6.3649) (0.5333, -6.384) (0.516, -6.423) (0.4981, -6.4618) (0.4887, -6.4815) (0.4693, -6.5216) (0.4492, -6.5615) (0.4388, -6.5817) (0.4172, -6.6228) (0.3948, -6.6636) (0.3833, -6.6843) (0.3594, -6.7263) (0.3349, -6.7678) (0.3222, -6.7889) (0.3013, -6.8229) (0.28, -6.8567) (0.2718, -6.8696) (0.2635, -6.8824) (0.2551, -6.8953) knots 0 0 0 0 0 0 0.004377 0.004377 0.004377 0.016733 0.016733 0.016733 0.036594 0.036594 0.036594 0.063277 0.063277 0.063277 0.096218 0.096218 0.096218 0.134948 0.134948 0.134948 0.179064 0.179064 0.179064 0.228222 0.228222 0.228222 0.282124 0.282124 0.282124 0.340507 0.340507 0.340507 0.403138 0.403138 0.403138 0.46981 0.46981 0.46981 0.540337 0.540337 0.540337 0.614551 0.614551 0.614551 0.692299 0.692299 0.692299 0.773444 0.773444 0.773444 0.857857 0.857857 0.857857 0.945422 0.945422 0.945422 1 1 1 1 1 1
  spline S39 degree 5 poles (-0.2551, -6.8953) (-0.2635, -6.8824) (-0.2718, -6.8696) (-0.28, -6.8567) (-0.3013, -6.8229) (-0.3222, -6.7889) (-0.3349, -6.7678) (-0.3594, -6.7263) (-0.3833, -6.6843) (-0.3948, -6.6636) (-0.4172, -6.6228) (-0.4388, -6.5817) (-0.4492, -6.5615) (-0.4693, -6.5216) (-0.4887, -6.4815) (-0.4981, -6.4618) (-0.516, -6.423) (-0.5333, -6.384) (-0.5415, -6.3649) (-0.5573, -6.3275) (-0.5725, -6.2898) (-0.5797, -6.2713) (-0.5934, -6.2353) (-0.6065, -6.1991) (-0.6127, -6.1815) (-0.6245, -6.1471) (-0.6356, -6.1126) (-0.6408, -6.0958) (-0.6506, -6.0632) (-0.6598, -6.0306) (-0.6641, -6.0147) (-0.6721, -5.9842) (-0.6795, -5.9536) (-0.683, -5.9389) (-0.6892, -5.9106) (-0.695, -5.8823) (-0.6976, -5.8687) (-0.7023, -5.843) (-0.7065, -5.8171) (-0.7083, -5.8049) (-0.7116, -5.7818) (-0.7144, -5.7588) (-0.7157, -5.7479) (-0.7177, -5.7279) (-0.7193, -5.7079) (-0.72, -5.6987) (-0.721, -5.6819) (-0.7216, -5.6652) (-0.7219, -5.6577) (-0.7221, -5.6447) (-0.7221, -5.6316) (-0.722, -5.6261) (-0.7218, -5.6169) (-0.7214, -5.6081) (-0.7211, -5.6042) (-0.7209, -5.6002) (-0.7204, -5.5948) (-0.7205, -5.5955) (-0.7199, -5.5908) (-0.7202, -5.5925) knots 0 0 0 0 0 0 0.054578 0.054578 0.054578 0.142143 0.142143 0.142143 0.226556 0.226556 0.226556 0.307701 0.307701 0.307701 0.385449 0.385449 0.385449 0.459663 0.459663 0.459663 0.53019 0.53019 0.53019 0.596862 0.596862 0.596862 0.659493 0.659493 0.659493 0.717876 0.717876 0.717876 0.771778 0.771778 0.771778 0.820936 0.820936 0.820936 0.865052 0.865052 0.865052 0.903782 0.903782 0.903782 0.936723 0.936723 0.936723 0.963406 0.963406 0.963406 0.983267 0.983267 0.983267 0.995623 0.995623 0.995623 1 1 1 1 1 1
  spline S40 degree 5 poles (-2.1726, -5.2033) (-2.1719, -5.2017) (-2.1738, -5.2061) (-2.1735, -5.2054) (-2.1758, -5.2104) (-2.1776, -5.2139) (-2.1793, -5.2174) (-2.1834, -5.2252) (-2.1878, -5.2334) (-2.1905, -5.2381) (-2.197, -5.2495) (-2.2037, -5.2607) (-2.2077, -5.2671) (-2.2166, -5.2812) (-2.2258, -5.2952) (-2.231, -5.3028) (-2.2424, -5.3194) (-2.2542, -5.3357) (-2.2607, -5.3444) (-2.2746, -5.363) (-2.289, -5.3813) (-2.2967, -5.391) (-2.3133, -5.4113) (-2.3302, -5.4312) (-2.3393, -5.4417) (-2.3584, -5.4634) (-2.378, -5.4847) (-2.3883, -5.4957) (-2.4101, -5.5186) (-2.4322, -5.541) (-2.4439, -5.5525) (-2.4682, -5.5762) (-2.4929, -5.5995) (-2.5059, -5.6114) (-2.5328, -5.6358) (-2.5601, -5.6597) (-2.5743, -5.6719) (-2.6037, -5.6967) (-2.6336, -5.721) (-2.6491, -5.7333) (-2.6811, -5.7584) (-2.7135, -5.7829) (-2.7302, -5.7954) (-2.7646, -5.8205) (-2.7995, -5.8451) (-2.8175, -5.8575) (-2.8544, -5.8826) (-2.8917, -5.907) (-2.9109, -5.9193) (-2.9502, -5.9441) (-2.9899, -5.9683) (-3.0102, -5.9804) (-3.0519, -6.0048) (-3.0939, -6.0285) (-3.1154, -6.0404) (-3.1505, -6.0595) (-3.1858, -6.078) (-3.1994, -6.0851) (-3.213, -6.0921) (-3.2267, -6.0991) knots 0 0 0 0 0 0 0.004377 0.004377 0.004377 0.016733 0.016733 0.016733 0.036594 0.036594 0.036594 0.063277 0.063277 0.063277 0.096218 0.096218 0.096218 0.134948 0.134948 0.134948 0.179064 0.179064 0.179064 0.228222 0.228222 0.228222 0.282124 0.282124 0.282124 0.340507 0.340507 0.340507 0.403138 0.403138 0.403138 0.46981 0.46981 0.46981 0.540337 0.540337 0.540337 0.614551 0.614551 0.614551 0.692299 0.692299 0.692299 0.773444 0.773444 0.773444 0.857857 0.857857 0.857857 0.945422 0.945422 0.945422 1 1 1 1 1 1
  spline S41 degree 5 poles (-3.6686, -5.8439) (-3.6694, -5.8286) (-3.6702, -5.8133) (-3.6708, -5.798) (-3.6724, -5.7581) (-3.6735, -5.7183) (-3.6739, -5.6937) (-3.6744, -5.6454) (-3.6741, -5.5971) (-3.6737, -5.5734) (-3.6727, -5.527) (-3.6708, -5.4805) (-3.6698, -5.4578) (-3.6673, -5.4132) (-3.664, -5.3688) (-3.6622, -5.347) (-3.6584, -5.3045) (-3.6538, -5.2621) (-3.6514, -5.2414) (-3.6464, -5.2011) (-3.6407, -5.1609) (-3.6377, -5.1413) (-3.6316, -5.1033) (-3.6248, -5.0653) (-3.6214, -5.0469) (-3.6144, -5.0113) (-3.6067, -4.9758) (-3.6028, -4.9587) (-3.5951, -4.9256) (-3.5867, -4.8927) (-3.5825, -4.8769) (-3.5742, -4.8465) (-3.5653, -4.8162) (-3.5609, -4.8017) (-3.5522, -4.7741) (-3.543, -4.7467) (-3.5385, -4.7337) (-3.5297, -4.709) (-3.5204, -4.6845) (-3.5159, -4.673) (-3.5072, -4.6514) (-3.4981, -4.63) (-3.4937, -4.62) (-3.4855, -4.6017) (-3.4769, -4.5835) (-3.4728, -4.5752) (-3.4654, -4.5602) (-3.4576, -4.5454) (-3.454, -4.5388) (-3.4477, -4.5274) (-3.4411, -4.5161) (-3.4383, -4.5113) (-3.4335, -4.5035) (-3.4288, -4.496) (-3.4266, -4.4928) (-3.4244, -4.4895) (-3.4213, -4.485) (-3.4217, -4.4856) (-3.4189, -4.4818) (-3.4199, -4.4832) knots 0 0 0 0 0 0 0.054578 0.054578 0.054578 0.142143 0.142143 0.142143 0.226556 0.226556 0.226556 0.307701 0.307701 0.307701 0.385449 0.385449 0.385449 0.459663 0.459663 0.459663 0.53019 0.53019 0.53019 0.596862 0.596862 0.596862 0.659493 0.659493 0.659493 0.717875 0.717875 0.717875 0.771778 0.771778 0.771778 0.820936 0.820936 0.820936 0.865052 0.865052 0.865052 0.903781 0.903781 0.903781 0.936723 0.936723 0.936723 0.963406 0.963406 0.963406 0.983267 0.983267 0.983267 0.995622 0.995622 0.995622 1 1 1 1 1 1
  spline S42 degree 5 poles (-4.4832, -3.4199) (-4.4818, -3.4189) (-4.4856, -3.4217) (-4.485, -3.4213) (-4.4895, -3.4244) (-4.4928, -3.4266) (-4.496, -3.4288) (-4.5035, -3.4335) (-4.5113, -3.4383) (-4.5161, -3.4411) (-4.5274, -3.4477) (-4.5388, -3.454) (-4.5454, -3.4576) (-4.5602, -3.4654) (-4.5752, -3.4728) (-4.5835, -3.4769) (-4.6017, -3.4855) (-4.62, -3.4937) (-4.63, -3.4981) (-4.6514, -3.5072) (-4.673, -3.5159) (-4.6845, -3.5204) (-4.709, -3.5297) (-4.7337, -3.5385) (-4.7467, -3.543) (-4.7741, -3.5522) (-4.8017, -3.5609) (-4.8162, -3.5653) (-4.8465, -3.5742) (-4.8769, -3.5825) (-4.8927, -3.5867) (-4.9256, -3.5951) (-4.9587, -3.6028) (-4.9758, -3.6067) (-5.0113, -3.6144) (-5.0469, -3.6214) (-5.0653, -3.6248) (-5.1033, -3.6316) (-5.1413, -3.6377) (-5.1609, -3.6407) (-5.2011, -3.6464) (-5.2414, -3.6514) (-5.2621, -3.6538) (-5.3045, -3.6584) (-5.347, -3.6622) (-5.3688, -3.664) (-5.4132, -3.6673) (-5.4578, -3.6698) (-5.4805, -3.6708) (-5.527, -3.6727) (-5.5734, -3.6737) (-5.5971, -3.6741) (-5.6454, -3.6744) (-5.6937, -3.6739) (-5.7183, -3.6735) (-5.7581, -3.6724) (-5.798, -3.6708) (-5.8133, -3.6702) (-5.8286, -3.6694) (-5.8439, -3.6686) knots 0 0 0 0 0 0 0.004377 0.004377 0.004377 0.016733 0.016733 0.016733 0.036594 0.036594 0.036594 0.063277 0.063277 0.063277 0.096218 0.096218 0.096218 0.134948 0.134948 0.134948 0.179064 0.179064 0.179064 0.228222 0.228222 0.228222 0.282124 0.282124 0.282124 0.340507 0.340507 0.340507 0.403138 0.403138 0.403138 0.46981 0.46981 0.46981 0.540337 0.540337 0.540337 0.614551 0.614551 0.614551 0.692299 0.692299 0.692299 0.773444 0.773444 0.773444 0.857857 0.857857 0.857857 0.945422 0.945422 0.945422 1 1 1 1 1 1
  spline S43 degree 5 poles (-6.0991, -3.2267) (-6.0921, -3.213) (-6.0851, -3.1994) (-6.078, -3.1858) (-6.0595, -3.1505) (-6.0404, -3.1154) (-6.0285, -3.0939) (-6.0048, -3.0519) (-5.9804, -3.0102) (-5.9683, -2.9899) (-5.9441, -2.9502) (-5.9193, -2.9109) (-5.907, -2.8917) (-5.8826, -2.8544) (-5.8575, -2.8175) (-5.8451, -2.7995) (-5.8205, -2.7646) (-5.7954, -2.7302) (-5.7829, -2.7135) (-5.7584, -2.6811) (-5.7333, -2.6491) (-5.721, -2.6336) (-5.6967, -2.6037) (-5.6719, -2.5743) (-5.6597, -2.5601) (-5.6358, -2.5328) (-5.6114, -2.5059) (-5.5995, -2.4929) (-5.5762, -2.4682) (-5.5525, -2.4439) (-5.541, -2.4322) (-5.5186, -2.4101) (-5.4957, -2.3883) (-5.4847, -2.378) (-5.4634, -2.3584) (-5.4417, -2.3393) (-5.4312, -2.3302) (-5.4113, -2.3133) (-5.391, -2.2967) (-5.3813, -2.289) (-5.363, -2.2746) (-5.3444, -2.2607) (-5.3357, -2.2542) (-5.3194, -2.2424) (-5.3028, -2.231) (-5.2952, -2.2258) (-5.2812, -2.2166) (-5.2671, -2.2077) (-5.2607, -2.2037) (-5.2495, -2.197) (-5.2381, -2.1905) (-5.2334, -2.1878) (-5.2252, -2.1834) (-5.2174, -2.1793) (-5.2139, -2.1776) (-5.2104, -2.1758) (-5.2054, -2.1735) (-5.2061, -2.1738) (-5.2017, -2.1719) (-5.2033, -2.1726) knots 0 0 0 0 0 0 0.054578 0.054578 0.054578 0.142143 0.142143 0.142143 0.226556 0.226556 0.226556 0.307701 0.307701 0.307701 0.385449 0.385449 0.385449 0.459663 0.459663 0.459663 0.53019 0.53019 0.53019 0.596862 0.596862 0.596862 0.659493 0.659493 0.659493 0.717876 0.717876 0.717876 0.771778 0.771778 0.771778 0.820936 0.820936 0.820936 0.865052 0.865052 0.865052 0.903782 0.903782 0.903782 0.936723 0.936723 0.936723 0.963406 0.963406 0.963406 0.983267 0.983267 0.983267 0.995623 0.995623 0.995623 1 1 1 1 1 1
  spline S44 degree 5 poles (-5.5925, -0.7202) (-5.5908, -0.7199) (-5.5955, -0.7205) (-5.5948, -0.7204) (-5.6002, -0.7209) (-5.6042, -0.7211) (-5.6081, -0.7214) (-5.6169, -0.7218) (-5.6261, -0.722) (-5.6316, -0.7221) (-5.6447, -0.7221) (-5.6577, -0.7219) (-5.6652, -0.7216) (-5.6819, -0.721) (-5.6987, -0.72) (-5.7079, -0.7193) (-5.7279, -0.7177) (-5.7479, -0.7157) (-5.7588, -0.7144) (-5.7818, -0.7116) (-5.8049, -0.7083) (-5.8171, -0.7065) (-5.843, -0.7023) (-5.8687, -0.6976) (-5.8823, -0.695) (-5.9106, -0.6892) (-5.9389, -0.683) (-5.9536, -0.6795) (-5.9842, -0.6721) (-6.0147, -0.6641) (-6.0306, -0.6598) (-6.0632, -0.6506) (-6.0958, -0.6408) (-6.1126, -0.6356) (-6.1471, -0.6245) (-6.1815, -0.6127) (-6.1991, -0.6065) (-6.2353, -0.5934) (-6.2713, -0.5797) (-6.2898, -0.5725) (-6.3275, -0.5573) (-6.3649, -0.5415) (-6.384, -0.5333) (-6.423, -0.516) (-6.4618, -0.4981) (-6.4815, -0.4887) (-6.5216, -0.4693) (-6.5615, -0.4492) (-6.5817, -0.4388) (-6.6228, -0.4172) (-6.6636, -0.3948) (-6.6843, -0.3833) (-6.7263, -0.3594) (-6.7678, -0.3349) (-6.7889, -0.3222) (-6.8229, -0.3013) (-6.8567, -0.28) (-6.8696, -0.2718) (-6.8824, -0.2635) (-6.8953, -0.2551) knots 0 0 0 0 0 0 0.004377 0.004377 0.004377 0.016733 0.016733 0.016733 0.036594 0.036594 0.036594 0.063277 0.063277 0.063277 0.096218 0.096218 0.096218 0.134948 0.134948 0.134948 0.179064 0.179064 0.179064 0.228222 0.228222 0.228222 0.282124 0.282124 0.282124 0.340507 0.340507 0.340507 0.403138 0.403138 0.403138 0.46981 0.46981 0.46981 0.540337 0.540337 0.540337 0.614551 0.614551 0.614551 0.692299 0.692299 0.692299 0.773444 0.773444 0.773444 0.857857 0.857857 0.857857 0.945422 0.945422 0.945422 1 1 1 1 1 1
  spline S45 degree 5 poles (-6.8953, 0.2551) (-6.8824, 0.2635) (-6.8696, 0.2718) (-6.8567, 0.28) (-6.8229, 0.3013) (-6.7889, 0.3222) (-6.7678, 0.3349) (-6.7263, 0.3594) (-6.6843, 0.3833) (-6.6636, 0.3948) (-6.6228, 0.4172) (-6.5817, 0.4388) (-6.5615, 0.4492) (-6.5216, 0.4693) (-6.4815, 0.4887) (-6.4618, 0.4981) (-6.423, 0.516) (-6.384, 0.5333) (-6.3649, 0.5415) (-6.3275, 0.5573) (-6.2898, 0.5725) (-6.2713, 0.5797) (-6.2353, 0.5934) (-6.1991, 0.6065) (-6.1815, 0.6127) (-6.1471, 0.6245) (-6.1126, 0.6356) (-6.0958, 0.6408) (-6.0632, 0.6506) (-6.0306, 0.6598) (-6.0147, 0.6641) (-5.9842, 0.6721) (-5.9536, 0.6795) (-5.9389, 0.683) (-5.9106, 0.6892) (-5.8823, 0.695) (-5.8687, 0.6976) (-5.843, 0.7023) (-5.8171, 0.7065) (-5.8049, 0.7083) (-5.7818, 0.7116) (-5.7588, 0.7144) (-5.7479, 0.7157) (-5.7279, 0.7177) (-5.7079, 0.7193) (-5.6987, 0.72) (-5.6819, 0.721) (-5.6652, 0.7216) (-5.6577, 0.7219) (-5.6447, 0.7221) (-5.6316, 0.7221) (-5.6261, 0.722) (-5.6169, 0.7218) (-5.6081, 0.7214) (-5.6042, 0.7211) (-5.6002, 0.7209) (-5.5948, 0.7204) (-5.5955, 0.7205) (-5.5908, 0.7199) (-5.5925, 0.7202) knots 0 0 0 0 0 0 0.054578 0.054578 0.054578 0.142143 0.142143 0.142143 0.226556 0.226556 0.226556 0.307701 0.307701 0.307701 0.385449 0.385449 0.385449 0.459663 0.459663 0.459663 0.53019 0.53019 0.53019 0.596862 0.596862 0.596862 0.659493 0.659493 0.659493 0.717876 0.717876 0.717876 0.771778 0.771778 0.771778 0.820936 0.820936 0.820936 0.865052 0.865052 0.865052 0.903782 0.903782 0.903782 0.936723 0.936723 0.936723 0.963406 0.963406 0.963406 0.983267 0.983267 0.983267 0.995623 0.995623 0.995623 1 1 1 1 1 1
  spline S46 degree 5 poles (-5.2033, 2.1726) (-5.2017, 2.1719) (-5.2061, 2.1738) (-5.2054, 2.1735) (-5.2104, 2.1758) (-5.2139, 2.1776) (-5.2174, 2.1793) (-5.2252, 2.1834) (-5.2334, 2.1878) (-5.2381, 2.1905) (-5.2495, 2.197) (-5.2607, 2.2037) (-5.2671, 2.2077) (-5.2812, 2.2166) (-5.2952, 2.2258) (-5.3028, 2.231) (-5.3194, 2.2424) (-5.3357, 2.2542) (-5.3444, 2.2607) (-5.363, 2.2746) (-5.3813, 2.289) (-5.391, 2.2967) (-5.4113, 2.3133) (-5.4312, 2.3302) (-5.4417, 2.3393) (-5.4634, 2.3584) (-5.4847, 2.378) (-5.4957, 2.3883) (-5.5186, 2.4101) (-5.541, 2.4322) (-5.5525, 2.4439) (-5.5762, 2.4682) (-5.5995, 2.4929) (-5.6114, 2.5059) (-5.6358, 2.5328) (-5.6597, 2.5601) (-5.6719, 2.5743) (-5.6967, 2.6037) (-5.721, 2.6336) (-5.7333, 2.6491) (-5.7584, 2.6811) (-5.7829, 2.7135) (-5.7954, 2.7302) (-5.8205, 2.7646) (-5.8451, 2.7995) (-5.8575, 2.8175) (-5.8826, 2.8544) (-5.907, 2.8917) (-5.9193, 2.9109) (-5.9441, 2.9502) (-5.9683, 2.9899) (-5.9804, 3.0102) (-6.0048, 3.0519) (-6.0285, 3.0939) (-6.0404, 3.1154) (-6.0595, 3.1505) (-6.078, 3.1858) (-6.0851, 3.1994) (-6.0921, 3.213) (-6.0991, 3.2267) knots 0 0 0 0 0 0 0.004377 0.004377 0.004377 0.016733 0.016733 0.016733 0.036594 0.036594 0.036594 0.063277 0.063277 0.063277 0.096218 0.096218 0.096218 0.134948 0.134948 0.134948 0.179064 0.179064 0.179064 0.228222 0.228222 0.228222 0.282124 0.282124 0.282124 0.340507 0.340507 0.340507 0.403138 0.403138 0.403138 0.46981 0.46981 0.46981 0.540337 0.540337 0.540337 0.614551 0.614551 0.614551 0.692299 0.692299 0.692299 0.773444 0.773444 0.773444 0.857857 0.857857 0.857857 0.945422 0.945422 0.945422 1 1 1 1 1 1
  spline S47 degree 5 poles (-5.8439, 3.6686) (-5.8286, 3.6694) (-5.8133, 3.6702) (-5.798, 3.6708) (-5.7581, 3.6724) (-5.7183, 3.6735) (-5.6937, 3.6739) (-5.6454, 3.6744) (-5.5971, 3.6741) (-5.5734, 3.6737) (-5.527, 3.6727) (-5.4805, 3.6708) (-5.4578, 3.6698) (-5.4132, 3.6673) (-5.3688, 3.664) (-5.347, 3.6622) (-5.3045, 3.6584) (-5.2621, 3.6538) (-5.2414, 3.6514) (-5.2011, 3.6464) (-5.1609, 3.6407) (-5.1413, 3.6377) (-5.1033, 3.6316) (-5.0653, 3.6248) (-5.0469, 3.6214) (-5.0113, 3.6144) (-4.9758, 3.6067) (-4.9587, 3.6028) (-4.9256, 3.5951) (-4.8927, 3.5867) (-4.8769, 3.5825) (-4.8465, 3.5742) (-4.8162, 3.5653) (-4.8017, 3.5609) (-4.7741, 3.5522) (-4.7467, 3.543) (-4.7337, 3.5385) (-4.709, 3.5297) (-4.6845, 3.5204) (-4.673, 3.5159) (-4.6514, 3.5072) (-4.63, 3.4981) (-4.62, 3.4937) (-4.6017, 3.4855) (-4.5835, 3.4769) (-4.5752, 3.4728) (-4.5602, 3.4654) (-4.5454, 3.4576) (-4.5388, 3.454) (-4.5274, 3.4477) (-4.5161, 3.4411) (-4.5113, 3.4383) (-4.5035, 3.4335) (-4.496, 3.4288) (-4.4928, 3.4266) (-4.4895, 3.4244) (-4.485, 3.4213) (-4.4856, 3.4217) (-4.4818, 3.4189) (-4.4832, 3.4199) knots 0 0 0 0 0 0 0.054578 0.054578 0.054578 0.142143 0.142143 0.142143 0.226556 0.226556 0.226556 0.307701 0.307701 0.307701 0.385449 0.385449 0.385449 0.459663 0.459663 0.459663 0.53019 0.53019 0.53019 0.596862 0.596862 0.596862 0.659493 0.659493 0.659493 0.717875 0.717875 0.717875 0.771778 0.771778 0.771778 0.820936 0.820936 0.820936 0.865052 0.865052 0.865052 0.903781 0.903781 0.903781 0.936723 0.936723 0.936723 0.963406 0.963406 0.963406 0.983267 0.983267 0.983267 0.995622 0.995622 0.995622 1 1 1 1 1 1
  point P0 (0, 0)
  dimension "d38" = 0.1
  measures "d38" radial gap between concentric circles of A10 A25
sketch "Sketch1" plane through (0, 0, 0) normal (0, 0, 1) x (1, 0, 0)
  arc A0 (-1.2609, -14.9469) -> (-1.2609, 14.9469) centre (0, 0) ccw
  arc A1 (-8.2391, 14.9469) -> (-8.2391, -14.9469) centre (-9.5, 0) ccw
  line L0 (-9.5, 0) -> (0, 0) construction
  arc A2 (-8.2391, 14.9469) -> (-1.2609, 14.9469) centre (-4.75, 56.3062) ccw
  arc A3 (-1.2609, -14.9469) -> (-8.2391, -14.9469) centre (-4.75, -56.3062) ccw
  circle A4 centre (-4.75, 0) radius 11.5
  line L1 (-24.5, 15) -> (15, 15) construction
  line L2 (15, 15) -> (15, -15) construction
  line L3 (15, -15) -> (-24.5, -15) construction
  line L4 (-24.5, -15) -> (-24.5, 15) construction
  dimension "d0" = 9.5
  dimension "d2" = 15
  dimension "d4" = 23
  dimension "d13" = 39.5
  dimension "d14" = 0.2
  constraints: 10 end point, 8 point on circle, 8 tangent, 5 centre point, 2 equal radius, 2 horizontal, 2 parallel, 1 coincident, 1 midpoint, 1 perpendicular
  measures "d0" distance of L0.start L0.end
  measures "d2" radius of A1
  measures "d4" diameter of A4
  measures "d13" distance between parallel lines of L2 L4
  measures "d14" distance edge to line of A2 L1
extrude "Extrusion1" add sketch "Sketch1" along normal mid plane 11
sketch "Sketch8" plane through (0, 0, 5.5) normal (0, 0, 1) x (1, 0, 0)
  arc A0 (-1.2609, -14.9469) -> (-1.2609, 14.9469) centre (0, 0) ccw construction
  arc A1 (-8.2391, 14.9469) -> (-1.2609, 14.9469) centre (-4.75, 56.3062) ccw construction
  arc A2 (-8.2391, 14.9469) -> (-8.2391, -14.9469) centre (-9.5, 0) ccw construction
  arc A3 (-1.2609, -14.9469) -> (-8.2391, -14.9469) centre (-4.75, -56.3062) ccw construction
  circle A4 centre (-4.75, 0) radius 11.5 construction
  arc A5 (-1.2021, -14.2494) -> (-1.2021, 14.2494) centre (0, 0) ccw
  arc A6 (-1.2021, -14.2494) -> (-8.2979, -14.2494) centre (-4.75, -56.3062) ccw
  arc A7 (-8.2979, 14.2494) -> (-8.2979, -14.2494) centre (-9.5, 0) ccw
  arc A8 (-8.2979, 14.2494) -> (-1.2021, 14.2494) centre (-4.75, 56.3062) ccw
  dimension "d27" = 0.7
  constraints: 8 point on circle, 4 centre point, 3 other
  measures "d27" radial gap between concentric circles of A0 A5
extrude "Extrusion7" cut sketch "Sketch8" against normal blind 0.3
mirror "Mirror1" about plane through (0, 0, 0) normal (0, 0, 1) of "Extrusion7"
chamfer "Chamfer1" distance 0.3 angle 45 8 edges at (14.3, 0, 5.5) (-4.75, -14.1, 5.5) (-23.8, 0, 5.5) (-4.75, 14.1, 5.5) (14.3, 0, -5.5) (-4.75, 14.1, -5.5) (-23.8, 0, -5.5) (-4.75, -14.1, -5.5)
sketch "Sketch12" plane through (-4.75, -56.3062, -5.2) normal (0, 0, -1) x (-1, 0, 0)
  circle A0 centre (0, 56.3062) radius 11.5 projected
  circle A1 centre (0, 56.3062) radius 7.5
  point P0 (-4.75, 56.3062)
  dimension "d42" = 15
  constraints: 1 centre point, 1 coincident
  measures "d42" diameter of A1
extrude "Extrusion11" add sketch "Sketch12" along normal blind 5 and the other way blind 2.5 contours A1
spur gear teeth "Spur Gear1" teeth 24 pitch diameter 9.6 tip diameter 10.251 root diameter 8.451 face width 2 trims to tip circle yes start plane through (-4.75, 0, -10.2) normal (0, 0, -1) x (-1, 0, 0)